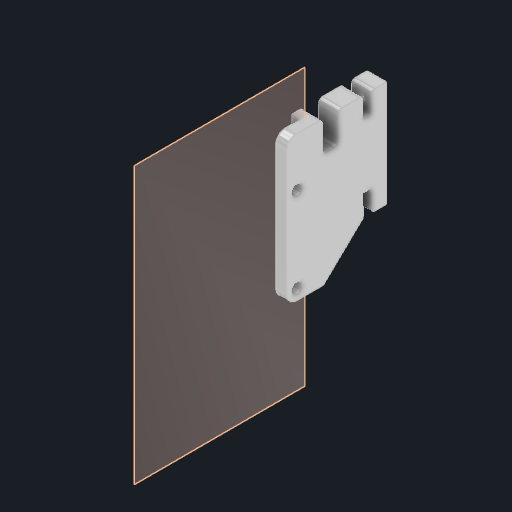
# Autodesk Inventor part: Dynamixel Vertical fixation
Saved by Autodesk Inventor 2024.3 (Build 283343000, 343)
## iProperties
Created: 2022-06-18
Part Number: Dynamixel Vertical fixation
Material: 알루미늄 6061
Document SubType Name: Sheet Metal
Designer: 박지훈
Density: 2.7 g/cm^3
Sheet Metal Rule: 기본값_mm
Appearance: 알루미늄 - 연마
Flat Pattern Width: 0.5 cm
Flat Pattern Length: 3.74 cm
Flat Pattern Area: 1.87 cm^2
Sheet Metal Width: 5.000 mm
Sheet Metal Length: 37.400 mm
Sheet Metal Area: 187.000 mm^2
Author: 박지훈
Autodesk Inventor part; units mm, degrees
ref_plane "YZ Plane" through (0, 0, 0) normal (1, 0, 0) x (0, 1, 0)
ref_plane "XZ Plane" through (0, 0, 0) normal (0, 1, 0) x (-1, 0, 0)
ref_plane "XY Plane" through (0, 0, 0) normal (0, 0, 1) x (1, 0, 0)
ref_plane "작업 평면1" through (19.4452, -233.7171, 54.1562) normal (1, 0, 0) x (0, 0, 1)
sketch "스케치1" plane through (19.4452, -233.7171, 54.1562) normal (1, 0, 0) x (0, 0, 1)
  line L0 (-15, 14.5) -> (-11.5, 14.5) projected
  line L1 (-15, 14.5) -> (-20.1, 8.5) projected
  line L2 (-20.1, 8.5) -> (-20.1, -44.6) projected
  line L3 (-20.1, -44.6) -> (-15, -50.6) projected
  line L4 (-15, -50.6) -> (15, -50.6) projected
  line L5 (15, -50.6) -> (20.1, -44.6) projected
  line L6 (20.1, -44.6) -> (20.1, 8.5) projected
  line L7 (20.1, 8.5) -> (15, 14.5) projected
  line L8 (11.5, 14.5) -> (15, 14.5) projected
  arc A0 (14.5, 11.5) -> (11.5, 14.5) centre (11.5, 11.5) ccw projected
  line L9 (14.5, -42) -> (14.5, 11.5) projected
  arc A1 (11.5, -45) -> (14.5, -42) centre (11.5, -42) ccw projected
  line L10 (-11.5, -45) -> (11.5, -45) projected
  arc A2 (-14.5, -42) -> (-11.5, -45) centre (-11.5, -42) ccw projected
  line L11 (-14.5, 11.5) -> (-14.5, -42) projected
  arc A3 (-11.5, 14.5) -> (-14.5, 11.5) centre (-11.5, 11.5) ccw projected
  circle A4 centre (-17.3, 4) radius 1.35 projected
  circle A5 centre (-17.3, -18) radius 1.35 projected
  circle A6 centre (-11, -47.8) radius 1.35 projected
  circle A7 centre (17.3, 4) radius 1.35 projected
  circle A8 centre (17.3, -18) radius 1.35 projected
  circle A9 centre (11, -47.8) radius 1.35 projected
  circle A10 centre (-17.3, -40) radius 1.35 projected
  circle A11 centre (17.3, -40) radius 1.35 projected
  line L12 (-14.9538, -50.5) -> (-20, -44.5632)
  line L13 (-20, 8.4632) -> (-14.9538, 14.4)
  line L14 (-14.9538, 14.4) -> (-12.5954, 14.4)
  arc A12 (-12.5954, 14.4) -> (-14.6, 11.5) centre (-11.5, 11.5) ccw
  line L15 (-14.6, 11.5) -> (-14.6, -42)
  arc A13 (-14.6, -42) -> (-11.5, -45.1) centre (-11.5, -42) ccw
  line L16 (-11.5, -45.1) -> (11.5, -45.1)
  arc A14 (11.5, -45.1) -> (14.6, -42) centre (11.5, -42) ccw
  line L17 (14.6, -42) -> (14.6, 11.5)
  arc A15 (14.6, 11.5) -> (12.5954, 14.4) centre (11.5, 11.5) ccw
  line L18 (12.5954, 14.4) -> (14.9538, 14.4)
  line L19 (14.9538, 14.4) -> (20, 8.4632)
  line L20 (20, 8.4632) -> (20, -44.5632)
  line L21 (20, -44.5632) -> (14.9538, -50.5)
  line L22 (14.9538, -50.5) -> (-14.9538, -50.5)
  arc A16 (-17.3, -42.7) -> (-14.6, -40) centre (-17.3, -40) ccw
  arc A17 (-14.6, -18) -> (-17.3, -15.3) centre (-17.3, -18) ccw
  line L23 (-17.3, -42.7) -> (-36.1, -42.7)
  line L24 (-36.1, -15.3) -> (-17.3, -15.3)
  line L25 (-36.1, -40) -> (-36.1, -37.3)
  line L26 (-36.1, -37.3) -> (-20.2, -37.3)
  line L27 (-36.1, -18) -> (-36.1, -20.7)
  line L28 (-20, -44.5632) -> (-20, -42.7)
  line L29 (-20, -15.3) -> (-20, 8.4632)
  line L30 (-36.1, -42.7) -> (-36.1, -37.3)
  line L31 (-36.1, -20.7) -> (-36.1, -15.3)
  line L32 (-20.2, -37.3) -> (-20.2, -20.7)
  line L33 (-36.1, -20.7) -> (-20.2, -20.7)
  point P0 (-36.1, -40)
  point P1 (-36.1, -18)
  dimension "d0" = 0.1
  dimension "d1" = 18.8
  dimension "d2" = 2.7
  dimension "d3" = 2.7
  constraints: 44 end point, 12 point on circle, 6 centre point, 4 point on line, 2 coincident, 2 perpendicular, 2 tangent, 1 horizontal, 1 parallel, 13 other
  measures "d0" distance between parallel lines of L3 L12
  measures "d1" distance of L24.end L24.start
  measures "d2" distance of L25.start L25.end
  measures "d3" distance of L27.end L27.start
extrude "돌출1" add sketch "스케치1" along normal blind 2.75 contours L24 A17 L15 A16 L23 L2 | L2 L23 L30 L25 L26 L32 L33 L27 L31 L24
sketch "스케치2" plane through (19.4452, -233.7171, 54.1562) normal (-1, 0, 0) x (0, 0, 1)
  line L0 (-36.1, 37.3) -> (-36.1, 42.7) projected
  line L1 (-20.2, 37.3) -> (-36.1, 37.3) projected
  line L2 (-20.2, 20.7) -> (-20.2, 37.3) projected
  line L3 (-36.1, 20.7) -> (-20.2, 20.7) projected
  line L4 (-36.1, 15.3) -> (-36.1, 20.7) projected
  line L5 (-17.3, 15.3) -> (-36.1, 15.3) projected
  arc A0 (-17.3, 15.3) -> (-14.6, 18) centre (-17.3, 18) ccw projected
  line L6 (-14.6, 40) -> (-14.6, 18) projected
  arc A1 (-14.6, 40) -> (-17.3, 42.7) centre (-17.3, 40) ccw projected
  line L7 (-36.1, 42.7) -> (-17.3, 42.7) projected
  circle A2 centre (-17.3, 40) radius 1.35 projected
  circle A3 centre (-17.3, 18) radius 1.35 projected
  line L8 (-36.1, 37.3) -> (-36.1, 42.7) projected
  line L9 (-36.1, 42.7) -> (-17.3, 42.7) projected
  line L10 (-36.1, 37.3) -> (-20.2, 37.3)
  line L11 (-20.2, 37.3) -> (-20.2, 42.7)
  line L12 (-20.2, 42.7) -> (-36.1, 42.7)
  line L13 (-36.1, 42.7) -> (-36.1, 37.3)
  line L14 (-36.1, 20.7) -> (-20.2, 20.7) projected
  line L15 (-17.3, 15.3) -> (-36.1, 15.3) projected
  line L16 (-20.2, 20.7) -> (-36.1, 20.7)
  line L17 (-36.1, 20.7) -> (-36.1, 15.3)
  line L18 (-36.1, 15.3) -> (-20.2, 15.3)
  line L19 (-20.2, 15.3) -> (-20.2, 20.7)
  point P0 (-20.2, 15.3)
  point P1 (-20.2, 37.3)
  point P2 (-20.2, 42.7)
  constraints: 16 end point, 4 parallel, 2 horizontal, 2 perpendicular, 1 point on line
extrude "돌출2" add sketch "스케치2" along normal blind 2.25 contours L0 L7 L11 L1 | L19 L5 L4 L3
sketch "스케치3" plane through (22.1952, -196.4171, 18.0562) normal (0, 0, -1) x (-1, 0, 0)
  line L0 (5, 5.4) -> (0, 5.4) projected
  line L1 (0, 0) -> (0, 5.4) projected
  line L2 (0, 0) -> (5, 0) projected
  line L3 (5, 5.4) -> (5, 0) projected
  line L4 (5, -16.6) -> (0, -16.6) projected
  line L5 (0, -22) -> (0, -16.6) projected
  line L6 (5, -22) -> (0, -22) projected
  line L7 (5, -16.6) -> (5, -22) projected
  line L8 (0, 0) -> (5, 0) projected
  line L9 (2.75, 2.7) -> (0, 2.7) projected
  line L10 (5, 0) -> (2.5, 0)
  line L11 (2.5, 0) -> (2.5, 2.7)
  line L12 (2.5, 2.7) -> (5, 2.7)
  line L13 (5, 2.7) -> (5, 0)
  circle A0 centre (2.5, 2.7) radius 1
  line L14 (2.75, -19.3) -> (0, -19.3) projected
  circle A1 centre (2.5, -19.3) radius 1
  dimension "d9" = 2
  dimension "d10" = 2
  constraints: 8 end point, 2 centre point, 2 parallel, 2 point on line, 1 coincident, 1 horizontal, 1 perpendicular
  measures "d9" diameter of A0
  measures "d10" diameter of A1
extrude "돌출3" cut sketch "스케치3" against normal blind 10 contours A0 L11 L9 L12 | L12 L9 A0 | L9 L11 A0 | A1
sketch "스케치4" plane through (22.1952, -196.4171, 18.0562) normal (0, 0, -1) x (-1, 0, 0)
  circle A0 centre (2.5, 2.7) radius 1 projected
  line L0 (5, 5.4) -> (0, 5.4) projected
  line L1 (0, 0) -> (0, 5.4) projected
  line L2 (0, 0) -> (5, 0) projected
  line L3 (5, 5.4) -> (5, 0) projected
  circle A1 centre (2.5, -19.3) radius 1 projected
  line L4 (5, -16.6) -> (0, -16.6) projected
  line L5 (0, -22) -> (0, -16.6) projected
  line L6 (5, -22) -> (0, -22) projected
  line L7 (5, -16.6) -> (5, -22) projected
extrude "돌출4" cut sketch "스케치4" against normal blind 1.7
sketch "스케치5" plane through (22.1952, -196.4171, 19.7562) normal (0, 0, -1) x (-1, 0, 0)
  line L0 (5, 5.4) -> (5, 0) projected
  line L1 (0, 5.4) -> (5, 5.4) projected
  line L2 (0, 0) -> (0, 5.4) projected
  line L3 (5, 0) -> (0, 0) projected
  circle A0 centre (2.5, 2.7) radius 1 projected
  line L4 (0, -16.6) -> (5, -16.6) projected
  line L5 (0, -22) -> (0, -16.6) projected
  line L6 (5, -22) -> (0, -22) projected
  line L7 (5, -16.6) -> (5, -22) projected
  circle A1 centre (2.5, -19.3) radius 1 projected
extrude "돌출5" add sketch "스케치5" along normal blind 0.6
sketch "스케치6" plane through (22.1952, -196.4171, 19.1562) normal (0, 0, -1) x (-1, 0, 0)
  line L0 (0, 5.4) -> (0, 0) projected
  line L1 (0, 0) -> (5, 0) projected
  line L2 (5, 0) -> (5, 5.4) projected
  line L3 (5, 5.4) -> (0, 5.4) projected
  circle A0 centre (2.5, 2.7) radius 1 projected
  line L4 (0, -22) -> (5, -22) projected
  line L5 (5, -22) -> (5, -16.6) projected
  line L6 (5, -16.6) -> (0, -16.6) projected
  line L7 (0, -16.6) -> (0, -22) projected
  circle A1 centre (2.5, -19.3) radius 1 projected
extrude "돌출6" cut sketch "스케치6" against normal blind 2.5 contours L3 L2 L1 L0 | A0 | L7 L6 L5 L4
sketch "스케치7" plane through (22.1952, -196.4171, 21.6562) normal (0, 0, -1) x (-1, 0, 0)
  line L0 (5, -16.6) -> (5, -22) projected
  line L1 (0, -16.6) -> (5, -16.6) projected
  line L2 (0, -22) -> (0, -16.6) projected
  line L3 (5, -22) -> (0, -22) projected
  circle A0 centre (2.5, -19.3) radius 1 projected
  circle A1 centre (2.5, 2.7) radius 1 projected
  line L4 (5, 0) -> (0, 0) projected
  line L5 (5, 5.4) -> (5, 0) projected
  line L6 (0, 5.4) -> (5, 5.4) projected
  line L7 (0, 0) -> (0, 5.4) projected
extrude "돌출7" add sketch "스케치7" along normal blind 0.2
sketch "스케치8" plane through (22.1952, -196.4171, 21.4562) normal (0, 0, -1) x (-1, 0, 0)
  line L0 (5, 5.4) -> (0, 5.4) projected
  line L1 (0, 5.4) -> (0, 0) projected
  line L2 (0, 0) -> (5, 0) projected
  line L3 (5, 0) -> (5, 5.4) projected
  circle A0 centre (2.5, 2.7) radius 1 projected
  line L4 (0, -16.6) -> (0, -22) projected
  line L5 (0, -22) -> (5, -22) projected
  line L6 (5, -22) -> (5, -16.6) projected
  line L7 (5, -16.6) -> (0, -16.6) projected
  circle A1 centre (2.5, -19.3) radius 1 projected
  point P0 (22.1952, 196.4171)
extrude "돌출8" add sketch "스케치8" along normal blind 1.3
move faces "이동1" translate (0, 0, -6.5) faces at (19.7354, -217.848, 20.1562) (19.7354, -191.5861, 20.1562)
sketch "스케치9" plane through (22.1952, -233.7171, 54.1562) normal (1, 0, 0) x (0, 0, -1)
  line L0 (40.5, 20.7) -> (20.2, 20.7) projected
  line L1 (20.2, 20.7) -> (20.2, 37.3) projected
  line L2 (20.2, 37.3) -> (40.5, 37.3) projected
  line L3 (40.5, 42.7) -> (40.5, 37.3) projected
  line L4 (40.5, 42.7) -> (17.3, 42.7) projected
  arc A0 (17.3, 42.7) -> (14.6, 40) centre (17.3, 40) ccw projected
  line L5 (14.6, 40) -> (14.6, 18) projected
  arc A1 (14.6, 18) -> (17.3, 15.3) centre (17.3, 18) ccw projected
  line L6 (17.3, 15.3) -> (40.5, 15.3) projected
  line L7 (40.5, 20.7) -> (40.5, 15.3) projected
  circle A2 centre (17.3, 40) radius 1.35 projected
  circle A3 centre (17.3, 18) radius 1.35 projected
  line L8 (40.5, 42.7) -> (40.5, 15.3)
  line L9 (30.5, 42.7) -> (30.5, 15.3)
  point P0 (54.1562, 233.7171)
  point P1 (30.5, 37.3)
  point P2 (30.5, 20.7)
  point P3 (40.5, 20.7)
  dimension "d26" = 10
  constraints: 4 end point, 1 collinear, 1 parallel
  measures "d26" distance between parallel lines of L8 L9
extrude "돌출9" add sketch "스케치9" against normal up to surface (5 mm away) contours L0 L9 L2 L8
sketch "스케치10" plane through (22.1952, -233.7171, 54.1562) normal (1, 0, 0) x (0, 0, -1)
  line L0 (30.5, 20.7) -> (20.2, 20.7) projected
  line L1 (20.2, 20.7) -> (20.2, 37.3) projected
  line L2 (20.2, 37.3) -> (30.5, 37.3) projected
  line L3 (30.5, 37.3) -> (30.5, 20.7) projected
  line L4 (40.5, 42.7) -> (40.5, 15.3) projected
  line L5 (40.5, 42.7) -> (17.3, 42.7) projected
  arc A0 (17.3, 42.7) -> (14.6, 40) centre (17.3, 40) ccw projected
  line L6 (14.6, 40) -> (14.6, 18) projected
  arc A1 (14.6, 18) -> (17.3, 15.3) centre (17.3, 18) ccw projected
  line L7 (17.3, 15.3) -> (40.5, 15.3) projected
  circle A2 centre (17.3, 40) radius 1.35 projected
  circle A3 centre (17.3, 18) radius 1.35 projected
  line L8 (40.5, 42.7) -> (40.5, 15.3)
  line L9 (40.5, 15.3) -> (30.5, 15.3)
  line L10 (30.5, 15.3) -> (30.5, 42.7)
  line L11 (30.5, 42.7) -> (40.5, 42.7)
  point P0 (54.1562, 233.7171)
  point P1 (30.5, 42.7)
  point P2 (30.5, 15.3)
  constraints: 8 end point, 3 equal length, 1 perpendicular
extrude "돌출10" cut sketch "스케치10" against normal through all contours L10 L7 A1 L6 A0 L5 L2 L1 L0
sketch "스케치11" plane through (22.1952, -233.7171, 54.1562) normal (1, 0, 0) x (0, 0, -1)
  line L0 (-15, 62.5) -> (-11.5, 62.5) projected
  line L1 (-15, 62.5) -> (-20.1, 56.5) projected
  line L2 (-20.1, 56.5) -> (-20.1, 3.4) projected
  line L3 (-20.1, 3.4) -> (-15, -2.6) projected
  line L4 (-15, -2.6) -> (15, -2.6) projected
  line L5 (15, -2.6) -> (20.1, 3.4) projected
  line L6 (20.1, 3.4) -> (20.1, 56.5) projected
  line L7 (20.1, 56.5) -> (15, 62.5) projected
  line L8 (11.5, 62.5) -> (15, 62.5) projected
  arc A0 (14.5, 59.5) -> (11.5, 62.5) centre (11.5, 59.5) ccw projected
  line L9 (14.5, 6) -> (14.5, 59.5) projected
  arc A1 (11.5, 3) -> (14.5, 6) centre (11.5, 6) ccw projected
  line L10 (-11.5, 3) -> (11.5, 3) projected
  arc A2 (-14.5, 6) -> (-11.5, 3) centre (-11.5, 6) ccw projected
  line L11 (-14.5, 59.5) -> (-14.5, 6) projected
  arc A3 (-11.5, 62.5) -> (-14.5, 59.5) centre (-11.5, 59.5) ccw projected
  circle A4 centre (17.3, 52) radius 1.35 projected
  circle A5 centre (17.3, 30) radius 1.35 projected
  circle A6 centre (17.3, 8) radius 1.35 projected
  circle A7 centre (11, 0.2) radius 1.35 projected
  circle A8 centre (-17.3, 52) radius 1.35 projected
  circle A9 centre (-17.3, 30) radius 1.35 projected
  circle A10 centre (-17.3, 8) radius 1.35 projected
  circle A11 centre (-11, 0.2) radius 1.35 projected
  line L12 (17.3, 30) -> (17.3, 8) construction
  line L13 (14.6, 30) -> (14.6, 8)
  line L14 (20, 8) -> (20, 30)
  arc A12 (20, 30) -> (14.6, 30) centre (17.3, 30) ccw
  arc A13 (14.6, 8) -> (20, 8) centre (17.3, 8) ccw
  line L15 (17.3, 32.7) -> (17.3, 5.3)
  line L16 (17.3, 5.3) -> (24.3, 5.3)
  line L17 (24.3, 5.3) -> (24.3, 32.7)
  line L18 (24.3, 32.7) -> (17.3, 32.7)
  line L19 (24.3, 32.7) -> (30.5, 42.7)
  line L20 (40.5, 15.3) -> (30.5, 15.3) projected
  line L21 (24.3, 5.3) -> (30.5, 15.3)
  line L22 (30.5, 42.7) -> (30.5, 15.3) projected
  line L23 (30.5, 15.3) -> (40.5, 15.3) projected
  line L24 (40.5, 42.7) -> (40.5, 15.3) projected
  line L25 (40.5, 42.7) -> (30.5, 42.7) projected
  point P0 (54.1562, 233.7171)
  point P1 (17.3, 19)
  point P2 (30.5, 42.7)
  dimension "d31" = 5.4
  dimension "d32" = 7
  constraints: 20 end point, 6 point on circle, 4 tangent, 3 parallel, 2 centre point, 1 midpoint, 1 perpendicular, 1 vertical
  measures "d31" diameter of A13
  measures "d32" distance of L16.end L15.end
extrude "돌출11" add sketch "스케치11" against normal blind 2.75 contours L16 A13 L14 A12 L18 L6 | L6 L18 L17 L16 | L15 A6 A5 A12 L14 A13 | A13 L13 A12 L15 A5 A6 | L17 L19 L22 L21
sketch "스케치12" plane through (19.4452, -233.7171, 54.1562) normal (-1, 0, 0) x (0, 0, 1)
  line L0 (-14.6, 8) -> (-14.6, 30) projected
  arc A0 (-14.6, 30) -> (-17.3, 32.7) centre (-17.3, 30) ccw projected
  line L1 (-17.3, 32.7) -> (-24.3, 32.7) projected
  line L2 (-24.3, 32.7) -> (-30.5, 42.7) projected
  line L3 (-30.5, 40.9682) -> (-30.5, 42.7) projected
  line L4 (-30.5, 40.9682) -> (-30.5, 39.0318) projected
  line L5 (-30.5, 18.9682) -> (-30.5, 39.0318) projected
  line L6 (-30.5, 18.9682) -> (-30.5, 17.0318) projected
  line L7 (-30.5, 15.3) -> (-30.5, 17.0318) projected
  line L8 (-30.5, 15.3) -> (-24.3, 5.3) projected
  line L9 (-24.3, 5.3) -> (-17.3, 5.3) projected
  arc A1 (-17.3, 5.3) -> (-14.6, 8) centre (-17.3, 8) ccw projected
  circle A2 centre (-17.3, 30) radius 1.35 projected
  circle A3 centre (-17.3, 8) radius 1.35 projected
  line L10 (13.5, 8.25) -> (11.5, 8.25) projected
  arc A4 (11.5, 8.25) -> (9.25, 6) centre (11.5, 6) ccw projected
  line L11 (9.25, 6) -> (9.25, 4) projected
  arc A5 (8.25, 3) -> (9.25, 4) centre (8.25, 4) ccw projected
  line L12 (8.25, 3) -> (-8.25, 3) projected
  arc A6 (-9.25, 4) -> (-8.25, 3) centre (-8.25, 4) ccw projected
  line L13 (-9.25, 4) -> (-9.25, 6) projected
  arc A7 (-9.25, 6) -> (-11.5, 8.25) centre (-11.5, 6) ccw projected
  line L14 (-11.5, 8.25) -> (-13.5, 8.25) projected
  arc A8 (-14.5, 9.25) -> (-13.5, 8.25) centre (-13.5, 9.25) ccw projected
  line L15 (-14.5, 9.25) -> (-14.5, 56.25) projected
  arc A9 (-13.5, 57.25) -> (-14.5, 56.25) centre (-13.5, 56.25) ccw projected
  line L16 (-13.5, 57.25) -> (-11.5, 57.25) projected
  arc A10 (-11.5, 57.25) -> (-9.25, 59.5) centre (-11.5, 59.5) ccw projected
  line L17 (-9.25, 59.5) -> (-9.25, 62.5) projected
  line L18 (-15, 62.5) -> (-9.25, 62.5) projected
  line L19 (-20.1, 56.5) -> (-15, 62.5) projected
  line L20 (-20.1, 3.4) -> (-20.1, 56.5) projected
  line L21 (-15, -2.6) -> (-20.1, 3.4) projected
  line L22 (15, -2.6) -> (-15, -2.6) projected
  line L23 (20.1, 3.4) -> (15, -2.6) projected
  line L24 (20.1, 56.5) -> (20.1, 3.4) projected
  line L25 (15, 62.5) -> (20.1, 56.5) projected
  line L26 (9.25, 62.5) -> (15, 62.5) projected
  line L27 (9.25, 62.5) -> (9.25, 59.5) projected
  arc A11 (9.25, 59.5) -> (11.5, 57.25) centre (11.5, 59.5) ccw projected
  line L28 (11.5, 57.25) -> (13.5, 57.25) projected
  arc A12 (14.5, 56.25) -> (13.5, 57.25) centre (13.5, 56.25) ccw projected
  line L29 (14.5, 56.25) -> (14.5, 9.25) projected
  arc A13 (13.5, 8.25) -> (14.5, 9.25) centre (13.5, 9.25) ccw projected
  circle A14 centre (17.3, 52) radius 1.35 projected
  circle A15 centre (17.3, 30) radius 1.35 projected
  circle A16 centre (11, 0.2) radius 1.35 projected
  circle A17 centre (-17.3, 52) radius 1.35 projected
  circle A18 centre (-17.3, 30) radius 1.35 projected
  circle A19 centre (-11, 0.2) radius 1.35 projected
  circle A20 centre (17.3, 8) radius 1.35 projected
  circle A21 centre (-17.3, 8) radius 1.35 projected
  line L30 (-21.1, 56.8676) -> (-15.4624, 63.5)
  line L31 (-15.4624, 63.5) -> (-8.25, 63.5)
  line L32 (-8.25, 63.5) -> (-8.25, 59.5)
  arc A22 (-11.5, 56.25) -> (-8.25, 59.5) centre (-11.5, 59.5) ccw
  line L33 (-11.5, 56.25) -> (-13.5, 56.25)
  line L34 (-13.5, 56.25) -> (-13.5, 9.25)
  line L35 (-13.5, 9.25) -> (-11.5, 9.25)
  arc A23 (-8.25, 6) -> (-11.5, 9.25) centre (-11.5, 6) ccw
  line L36 (-8.25, 6) -> (-8.25, 4)
  line L37 (-8.25, 4) -> (8.25, 4)
  line L38 (8.25, 4) -> (8.25, 6)
  arc A24 (11.5, 9.25) -> (8.25, 6) centre (11.5, 6) ccw
  line L39 (11.5, 9.25) -> (13.5, 9.25)
  line L40 (13.5, 9.25) -> (13.5, 56.25)
  line L41 (13.5, 56.25) -> (11.5, 56.25)
  arc A25 (8.25, 59.5) -> (11.5, 56.25) centre (11.5, 59.5) ccw
  line L42 (8.25, 59.5) -> (8.25, 63.5)
  line L43 (8.25, 63.5) -> (15.4624, 63.5)
  line L44 (15.4624, 63.5) -> (21.1, 56.8676)
  line L45 (21.1, 56.8676) -> (21.1, 3.0324)
  line L46 (21.1, 3.0324) -> (15.4624, -3.6)
  line L47 (15.4624, -3.6) -> (-15.4624, -3.6)
  line L48 (-15.4624, -3.6) -> (-21.1, 3.0324)
  line L49 (-21.1, 3.0324) -> (-21.1, 56.8676)
  point P0 (-54.1562, 233.7171)
  point P1 (-21.1, 5.3)
  point P2 (-21.1, 32.7)
  dimension "d35" = 1
  constraints: 40 end point, 8 point on circle, 4 centre point, 23 other
  measures "d35" distance between parallel lines of L20 L49
extrude "돌출12" add sketch "스케치12" along normal up to surface (2.25 mm away) contours L9 L8 L7 L6 L5 L4 L3 L2 L1 L49
fillet "모깎기1" radius 5 3 edges at (19.6952, -218.4171, 23.6562) (19.6952, -191.0171, 23.6562) (19.6952, -201.0171, 29.8562)
sketch "스케치13" plane through (22.1952, -233.7171, 54.1562) normal (1, 0, 0) x (0, 0, -1)
  arc A0 (33.283, 42.7) -> (29.0335, 40.3347) centre (33.283, 37.7) ccw projected
  line L0 (29.0335, 40.3347) -> (25.7665, 35.0653) projected
  arc A1 (21.517, 32.7) -> (25.7665, 35.0653) centre (21.517, 37.7) ccw projected
  line L1 (21.517, 32.7) -> (17.3, 32.7) projected
  arc A2 (17.3, 32.7) -> (14.6, 30) centre (17.3, 30) ccw projected
  line L2 (14.6, 30) -> (14.6, 8) projected
  arc A3 (14.6, 8) -> (17.3, 5.3) centre (17.3, 8) ccw projected
  line L3 (17.3, 5.3) -> (24.3, 5.3) projected
  line L4 (24.3, 5.3) -> (29.0335, 12.9347) projected
  arc A4 (33.283, 15.3) -> (29.0335, 12.9347) centre (33.283, 10.3) ccw projected
  line L5 (33.283, 15.3) -> (40.5, 15.3) projected
  line L6 (40.5, 42.7) -> (40.5, 15.3) projected
  line L7 (40.5, 42.7) -> (33.283, 42.7) projected
  circle A5 centre (17.3, 30) radius 1.35 projected
  circle A6 centre (17.3, 8) radius 1.35 projected
  line L8 (30.8659, 31.9037) -> (33.8396, 36.7)
  line L9 (33.8396, 36.7) -> (34.5, 36.7)
  line L10 (34.5, 36.7) -> (34.5, 21.3)
  line L11 (34.5, 21.3) -> (33.283, 21.3)
  arc A7 (33.283, 21.3) -> (23.9341, 16.0963) centre (33.283, 10.3) ccw
  line L12 (23.9341, 16.0963) -> (20.9604, 11.3)
  line L13 (20.9604, 11.3) -> (20.6, 11.3)
  line L14 (20.6, 11.3) -> (20.6, 26.7)
  line L15 (20.6, 26.7) -> (21.517, 26.7)
  arc A8 (21.517, 26.7) -> (30.8659, 31.9037) centre (21.517, 37.7) ccw
  point P0 (54.1562, 233.7171)
  dimension "d39" = 6
  constraints: 16 end point, 4 point on circle, 2 centre point, 9 other
  measures "d39" radial gap between concentric circles of A1 A8
extrude "돌출13" cut sketch "스케치13" against normal through all contours L8 L9 L10 L11 A7 L12 L13 L14 L15 A8
fillet "모깎기2" radius 1 6 edges at (19.6952, -197.0171, 19.6562) (19.6952, -197.0171, 20.3166) (19.6952, -212.4171, 19.6562) (20.8202, -222.4171, 33.1958) (20.8202, -222.4171, 33.5562) (20.8202, -207.0171, 33.5562)
sketch "스케치14" plane through (22.1952, -233.7171, 54.1562) normal (1, 0, 0) x (0, 0, -1)
  line L0 (34.5, 34.2545) -> (34.5, 22.3) projected
  arc A0 (33.5, 21.3) -> (34.5, 22.3) centre (33.5, 22.3) ccw projected
  line L1 (33.5, 21.3) -> (33.283, 21.3) projected
  arc A1 (33.283, 21.3) -> (23.9341, 16.0963) centre (33.283, 10.3) ccw projected
  line L2 (23.9341, 16.0963) -> (22.4499, 13.7025) projected
  arc A2 (20.6, 14.2294) -> (22.4499, 13.7025) centre (21.6, 14.2294) ccw projected
  line L3 (20.6, 14.2294) -> (20.6, 25.7003) projected
  arc A3 (21.5931, 26.7003) -> (20.6, 25.7003) centre (21.6, 25.7003) ccw projected
  arc A4 (21.5931, 26.7003) -> (30.8659, 31.9037) centre (21.517, 37.7) ccw projected
  line L4 (30.8659, 31.9037) -> (32.6501, 34.7814) projected
  arc A5 (34.5, 34.2545) -> (32.6501, 34.7814) centre (33.5, 34.2545) ccw projected
  arc A6 (33.283, 42.7) -> (29.0335, 40.3347) centre (33.283, 37.7) ccw projected
  line L5 (29.0335, 40.3347) -> (25.7665, 35.0653) projected
  arc A7 (21.517, 32.7) -> (25.7665, 35.0653) centre (21.517, 37.7) ccw projected
  line L6 (21.517, 32.7) -> (17.3, 32.7) projected
  arc A8 (17.3, 32.7) -> (14.6, 30) centre (17.3, 30) ccw projected
  line L7 (14.6, 30) -> (14.6, 8) projected
  arc A9 (14.6, 8) -> (17.3, 5.3) centre (17.3, 8) ccw projected
  line L8 (17.3, 5.3) -> (24.3, 5.3) projected
  line L9 (24.3, 5.3) -> (29.0335, 12.9347) projected
  arc A10 (33.283, 15.3) -> (29.0335, 12.9347) centre (33.283, 10.3) ccw projected
  line L10 (33.283, 15.3) -> (40.5, 15.3) projected
  line L11 (40.5, 42.7) -> (40.5, 15.3) projected
  line L12 (40.5, 42.7) -> (33.283, 42.7) projected
  circle A11 centre (17.3, 30) radius 1.35 projected
  circle A12 centre (17.3, 8) radius 1.35 projected
  line L13 (14.6, 30) -> (14.6, 8) projected
  line L14 (14.6, 30) -> (40.5, 30)
  line L15 (40.5, 30) -> (40.5, 42.7)
  line L16 (40.5, 42.7) -> (14.6, 42.7)
  line L17 (14.6, 42.7) -> (14.6, 30)
  line L18 (24.3, 5.3) -> (40.5, 5.3)
  line L19 (40.5, 5.3) -> (40.5, 15.3)
  line L20 (40.5, 15.3) -> (24.3, 15.3)
  line L21 (24.3, 15.3) -> (24.3, 5.3)
  point P0 (54.1562, 233.7171)
  constraints: 16 end point, 4 parallel, 2 horizontal, 2 perpendicular
extrude "돌출14" add sketch "스케치14" against normal up to surface (2.75 mm away) contours L0 L14 A4 L4 A5 | L0 A0 L1 A1 L2 A2 L3 A3 A4 L14 | L19 L18 L9 A10 L10 | A6 L5 A7 L6 A8 L17 L16
sketch "스케치15" plane through (19.4452, -228.4171, 13.6562) normal (-1, 0, 0) x (0, 0, 1)
  arc A0 (11.4665, 7.6347) -> (7.217, 10) centre (7.217, 5) ccw projected
  line L0 (0, 10) -> (7.217, 10) projected
  line L1 (0, 10) -> (0, 0) projected
  line L2 (0, 0) -> (16.2, 0) projected
  line L3 (11.4665, 7.6347) -> (16.2, 0) projected
  line L4 (0, 37.4) -> (25.9, 37.4) projected
  line L5 (25.9, 37.4) -> (25.9, 2.7) projected
  arc A1 (23.2, 0) -> (25.9, 2.7) centre (23.2, 2.7) ccw projected
  line L6 (23.2, 0) -> (0, 0) projected
  line L7 (0, 37.4) -> (0, 0) projected
  circle A2 centre (23.2, 24.7) radius 1.35 projected
  circle A3 centre (23.2, 2.7) radius 1.35 projected
  line L8 (19.4, 8.0634) -> (19.4, 0) projected
  line L9 (19.4, 0) -> (23.2, 0) projected
  arc A4 (23.2, 0) -> (25.9, 2.7) centre (23.2, 2.7) ccw projected
  line L10 (25.9, 2.7) -> (25.9, 37.4) projected
  line L11 (25.9, 37.4) -> (7.217, 37.4) projected
  arc A5 (11.4665, 35.0347) -> (7.217, 37.4) centre (7.217, 32.4) ccw projected
  line L12 (14.7335, 29.7653) -> (11.4665, 35.0347) projected
  arc A6 (14.7335, 29.7653) -> (18.983, 27.4) centre (18.983, 32.4) ccw projected
  line L13 (19.4, 27.4) -> (18.983, 27.4) projected
  line L14 (19.4, 27.4) -> (19.4, 21.2663) projected
  arc A7 (19.4, 21.2663) -> (18.9069, 21.4003) centre (18.9, 20.4003) ccw projected
  arc A8 (18.0501, 8.4025) -> (19.4, 8.0634) centre (18.9, 8.9294) ccw projected
  circle A9 centre (23.2, 2.7) radius 1.35 projected
  circle A10 centre (23.2, 24.7) radius 1.35 projected
  line L15 (19.4, 8.0634) -> (19.4, 0) projected
  line L16 (0, 37.4) -> (25.9, 37.4) projected
  line L17 (19.4, 0) -> (25.9, 0)
  line L18 (25.9, 0) -> (25.9, 37.4)
  line L19 (25.9, 37.4) -> (19.4, 37.4)
  line L20 (19.4, 37.4) -> (19.4, 0)
  arc A11 (9.6341, 26.6037) -> (18.9069, 21.4003) centre (18.983, 32.4) ccw projected
  line L21 (7.8499, 29.4814) -> (9.6341, 26.6037) projected
  arc A12 (7.8499, 29.4814) -> (6, 28.9545) centre (7, 28.9545) ccw projected
  line L22 (6, 17) -> (6, 28.9545) projected
  arc A13 (6, 17) -> (7, 16) centre (7, 17) ccw projected
  line L23 (7.217, 16) -> (7, 16) projected
  arc A14 (16.5659, 10.7963) -> (7.217, 16) centre (7.217, 5) ccw projected
  line L24 (18.0501, 8.4025) -> (16.5659, 10.7963) projected
  point P0 (-13.6562, 228.4171)
  point P1 (19.4, 37.4)
  point P2 (7.217, 37.4)
  constraints: 8 end point, 2 parallel, 1 horizontal, 1 perpendicular
extrude "돌출15" add sketch "스케치15" along normal up to surface (2.25 mm away) contours L3 L2 L1 L0 A0 | A8 L24 A14 L23 A13 L22 A12 L21 A11 A7 L20 | L4 L20 L13 A6 L12 A5
fillet "모깎기3" radius 2.5 1 edges at (20.8202, -191.0171, 39.5562)
sketch "스케치16" plane through (22.1952, -233.7171, 54.1562) normal (1, 0, 0) x (0, 0, -1)
  circle A0 centre (17.3, 8) radius 1.35 projected
  circle A1 centre (17.3, 30) radius 1.35 projected
  arc A2 (17.1, 42.7) -> (14.6, 40.2) centre (17.1, 40.2) ccw projected
  line L0 (14.6, 40.2) -> (14.6, 8) projected
  arc A3 (14.6, 8) -> (17.3, 5.3) centre (17.3, 8) ccw projected
  line L1 (17.3, 5.3) -> (40.5, 5.3) projected
  line L2 (40.5, 42.7) -> (40.5, 5.3) projected
  line L3 (40.5, 42.7) -> (17.1, 42.7) projected
  line L4 (24.5, 46.4593) -> (24.5, 81.4701) projected
  line L5 (27.5, 81.4701) -> (27.5, 46.4593) projected
  line L6 (24.5, 81.4701) -> (27.5, 81.4701)
  line L7 (27.5, 81.4701) -> (27.5, 42.7)
  line L8 (27.5, 42.7) -> (24.5, 42.7)
  line L9 (24.5, 42.7) -> (24.5, 81.4701)
  line L10 (24.5, 42.7) -> (27.5, 42.7)
  line L11 (27.5, 42.7) -> (27.5, 36.7)
  line L12 (27.5, 36.7) -> (24.5, 36.7)
  line L13 (24.5, 36.7) -> (24.5, 42.7)
  point P0 (54.1562, 233.7171)
  point P1 (27.5, 42.7)
  point P2 (24.5, 42.7)
  dimension "d48" = 6
  constraints: 16 end point, 4 parallel, 2 perpendicular, 1 collinear, 1 horizontal
  measures "d48" distance of L7.end L11.end
extrude "돌출16" cut sketch "스케치16" against normal through all contours L3 L11 L12 L13
sketch "스케치17" plane through (22.1952, -197.0171, 26.6562) normal (0, 0, 1) x (1, 0, 0)
  circle A0 centre (-19.8, 11.3) radius 5 projected
  line L0 (-13.5254, 9.7593) -> (-4.9287, 44.7701) projected
  line L1 (-34.6713, 44.7701) -> (-26.0746, 9.7593) projected
  line L2 (-13.5254, 9.7593) -> (-4.9287, 44.7701)
  line L3 (-34.6713, 44.7701) -> (-26.0746, 9.7593)
  line L4 (-53.2701, -3.5713) -> (-18.2593, 5.0254)
  line L5 (-18.2593, 17.5746) -> (-53.2701, 26.1713)
  line L6 (-4.9287, -22.1701) -> (-13.5254, 12.8407)
  line L7 (-26.0746, 12.8407) -> (-34.6713, -22.1701)
  line L8 (13.6701, 26.1713) -> (-21.3407, 17.5746)
  line L9 (-21.3407, 5.0254) -> (13.6701, -3.5713)
  line L10 (-21.5792, 4.0542) -> (13.4317, -4.5425)
  circle A1 centre (-2.5, 3.3) radius 1 projected
  line L11 (-5, -31.4) -> (-5, 6) projected
  line L12 (-5, 6) -> (0, 6) projected
  line L13 (0, 6) -> (0, -31.4) projected
  line L14 (0, -31.4) -> (-5, -31.4) projected
  circle A2 centre (-2.5, -18.7) radius 1 projected
  line L15 (-5, 6) -> (0, 6)
  line L16 (0, 6) -> (0, -1.5)
  line L17 (0, -1.5) -> (-5, -1.5)
  line L18 (-5, -1.5) -> (-5, 6)
  point P0 (-22.1952, 197.0171)
  point P1 (-18.2593, 17.5746)
  point P2 (-53.2701, 26.1713)
  point P3 (-53.2701, -3.5713)
  point P4 (-18.2593, 5.0254)
  point P5 (-26.0746, 12.8407)
  point P6 (-34.6713, -22.1701)
  point P7 (-4.9287, -22.1701)
  point P8 (-13.5254, 12.8407)
  point P9 (-21.3407, 5.0254)
  point P10 (13.6701, -3.5713)
  point P11 (13.6701, 26.1713)
  point P12 (-21.3407, 17.5746)
  dimension "d53" = 360
  dimension "d55" = 1
  dimension "d56" = 7.5
  constraints: 26 end point, 4 equal length, 2 coincident, 1 perpendicular, 43 other
  measures "d55" distance between parallel lines of L9 L10
  measures "d56" distance of L12.end L16.end
extrude "돌출17" cut sketch "스케치17" along normal up to surface (3 mm away) contours L11 L12 L13 L9 | L9 L13 L10 L11 | L10 L13 L17 L11
sketch "스케치18" plane through (22.1952, -233.7171, 54.1562) normal (1, 0, 0) x (0, 0, -1)
  circle A0 centre (17.3, 8) radius 1.35 projected
  circle A1 centre (17.3, 30) radius 1.35 projected
  line L0 (27.5, 42.7) -> (27.5, 35.2) projected
  line L1 (27.5, 35.2) -> (24.5, 35.2) projected
  line L2 (24.5, 35.2) -> (24.5, 42.7) projected
  line L3 (24.5, 42.7) -> (17.1, 42.7) projected
  arc A2 (17.1, 42.7) -> (14.6, 40.2) centre (17.1, 40.2) ccw projected
  line L4 (14.6, 40.2) -> (14.6, 8) projected
  arc A3 (14.6, 8) -> (17.3, 5.3) centre (17.3, 8) ccw projected
  line L5 (17.3, 5.3) -> (40.5, 5.3) projected
  line L6 (40.5, 42.7) -> (40.5, 5.3) projected
  line L7 (40.5, 42.7) -> (27.5, 42.7) projected
  line L8 (28, 34.7) -> (28, 42.2)
  line L9 (28, 42.2) -> (40, 42.2)
  line L10 (40, 42.2) -> (40, 5.8)
  line L11 (40, 5.8) -> (17.3, 5.8)
  arc A4 (15.1, 8) -> (17.3, 5.8) centre (17.3, 8) ccw
  line L12 (15.1, 8) -> (15.1, 40.2)
  arc A5 (17.1, 42.2) -> (15.1, 40.2) centre (17.1, 40.2) ccw
  line L13 (17.1, 42.2) -> (24, 42.2)
  line L14 (24, 42.2) -> (24, 34.7)
  line L15 (24, 34.7) -> (28, 34.7)
  line L16 (24, 42.2) -> (28, 42.2)
  line L17 (28, 42.2) -> (28, 42.7)
  line L18 (28, 42.7) -> (24, 42.7)
  line L19 (24, 42.7) -> (24, 42.2)
  point P0 (54.1562, 233.7171)
  point P1 (27.5, 42.7)
  point P2 (24, 42.7)
  point P3 (28, 42.7)
  point P4 (27.5, 42.2)
  point P5 (24.5, 42.2)
  dimension "d59" = 0.5
  constraints: 24 end point, 4 point on circle, 2 centre point, 2 parallel, 2 perpendicular, 9 other
  measures "d59" distance between parallel lines of L0 L8
extrude "돌출18" cut sketch "스케치18" against normal through all contours L7 L17 L16 L0 | L0 L16 L2 L18 | L16 L8 L15 L14 L2 L1 L0 | L2 L16 L19 L3
fillet "모깎기4" radius 1 4 edges at (19.6952, -191.0171, 26.1562) (19.6952, -191.0171, 30.1562) (19.6952, -199.0171, 30.1562) (19.6952, -199.0171, 26.1562)
sketch "스케치19" plane through (22.1952, -233.7171, 54.1562) normal (1, 0, 0) x (0, 0, -1)
  arc A0 (24, 41.7) -> (23, 42.7) centre (23, 41.7) ccw projected
  line L0 (23, 42.7) -> (17.1, 42.7) projected
  arc A1 (17.1, 42.7) -> (14.6, 40.2) centre (17.1, 40.2) ccw projected
  line L1 (14.6, 40.2) -> (14.6, 8) projected
  arc A2 (14.6, 8) -> (17.3, 5.3) centre (17.3, 8) ccw projected
  line L2 (17.3, 5.3) -> (40.5, 5.3) projected
  line L3 (40.5, 42.7) -> (40.5, 5.3) projected
  line L4 (40.5, 42.7) -> (29, 42.7) projected
  arc A3 (29, 42.7) -> (28, 41.7) centre (29, 41.7) ccw projected
  line L5 (28, 41.7) -> (28, 35.7) projected
  arc A4 (27, 34.7) -> (28, 35.7) centre (27, 35.7) ccw projected
  line L6 (27, 34.7) -> (25, 34.7) projected
  arc A5 (24, 35.7) -> (25, 34.7) centre (25, 35.7) ccw projected
  line L7 (24, 35.7) -> (24, 41.7) projected
  circle A6 centre (17.3, 30) radius 1.35 projected
  circle A7 centre (17.3, 8) radius 1.35 projected
  line L8 (40.5, 38.65) -> (40.5, 41.35) projected
  line L9 (40.5, 16.65) -> (40.5, 19.35) projected
  line L10 (40.5, 19) -> (40.5, 17) projected
  line L11 (40.5, 18) -> (40.5, 15.3)
  line L12 (40.5, 18) -> (43.2, 18) construction
  line L13 (40.5, 15.3) -> (21.1, 5.3)
  line L14 (17.3, 5.3) -> (40.5, 5.3) projected
  arc A8 (17.1, 42.7) -> (14.6, 40.2) centre (17.1, 40.2) ccw projected
  line L15 (17.1, 42.7) -> (21.1, 42.7) projected
  line L16 (21.1, 42.7) -> (21.1, 5.3) projected
  line L17 (21.1, 5.3) -> (17.3, 5.3) projected
  arc A9 (14.6, 8) -> (17.3, 5.3) centre (17.3, 8) ccw projected
  line L18 (14.6, 8) -> (14.6, 40.2) projected
  circle A10 centre (17.3, 30) radius 1.35 projected
  circle A11 centre (17.3, 8) radius 1.35 projected
  line L19 (40.5, 15.3) -> (37.5, 15.3)
  line L20 (37.5, 15.3) -> (21.1, 5.3)
  line L21 (21.1, 5.3) -> (24.1, 5.3)
  line L22 (24.1, 5.3) -> (37.5, 15.3)
  point P0 (54.1562, 233.7171)
  point P1 (40.5, 15.3)
  dimension "d63" = 2.7
  dimension "d64" = 90
  dimension "d65" = 3
  dimension "d66" = 3
  constraints: 14 end point, 2 perpendicular, 2 point on line, 1 collinear, 1 horizontal, 1 midpoint
  measures "d63" distance of L11.start L11.end
  measures "d64" angle of L11 L12
  measures "d65" distance of L11.end L19.end
  measures "d66" distance of L13.end L21.end
extrude "돌출19" cut sketch "스케치19" against normal through all contours L22 L13 L3 L2 | L22 L19 L13
sketch "스케치20" plane through (22.1952, -233.7171, 54.1562) normal (1, 0, 0) x (0, 0, -1)
  line L0 (40.5, 41) -> (40.5, 39) projected
  line L1 (40.5, 16.65) -> (40.5, 19.35) projected
  line L2 (40.5, 40) -> (40.5, 18)
  line L3 (40.5, 18) -> (35.5, 18)
  line L4 (35.5, 18) -> (35.5, 40)
  line L5 (35.5, 40) -> (40.5, 40)
  line L6 (29, 42.7) -> (40.5, 42.7) projected
  line L7 (34.5, 37.3) -> (36.5, 37.3)
  line L8 (36.5, 37.3) -> (36.5, 42.7)
  line L9 (36.5, 42.7) -> (34.5, 42.7)
  line L10 (34.5, 42.7) -> (34.5, 37.3)
  line L11 (34.5, 37.3) -> (36.5, 42.7) construction
  line L12 (36.5, 37.3) -> (34.5, 42.7) construction
  line L13 (36.5, 20.7) -> (34.5, 20.7)
  line L14 (34.5, 20.7) -> (34.5, 15.3)
  line L15 (34.5, 15.3) -> (36.5, 15.3)
  line L16 (36.5, 15.3) -> (36.5, 20.7)
  line L17 (36.5, 20.7) -> (34.5, 15.3) construction
  line L18 (34.5, 20.7) -> (36.5, 15.3) construction
  circle A0 centre (17.3, 8) radius 1.35 projected
  circle A1 centre (17.3, 30) radius 1.35 projected
  line L19 (24.1, 5.3) -> (37.5, 15.3) projected
  line L20 (37.5, 15.3) -> (40.5, 15.3) projected
  line L21 (40.5, 42.7) -> (40.5, 15.3) projected
  line L22 (40.5, 42.7) -> (29, 42.7) projected
  arc A2 (29, 42.7) -> (28, 41.7) centre (29, 41.7) ccw projected
  line L23 (28, 41.7) -> (28, 35.7) projected
  arc A3 (27, 34.7) -> (28, 35.7) centre (27, 35.7) ccw projected
  line L24 (27, 34.7) -> (25, 34.7) projected
  arc A4 (24, 35.7) -> (25, 34.7) centre (25, 35.7) ccw projected
  line L25 (24, 35.7) -> (24, 41.7) projected
  arc A5 (24, 41.7) -> (23, 42.7) centre (23, 41.7) ccw projected
  line L26 (23, 42.7) -> (17.1, 42.7) projected
  arc A6 (17.1, 42.7) -> (14.6, 40.2) centre (17.1, 40.2) ccw projected
  line L27 (14.6, 40.2) -> (14.6, 8) projected
  arc A7 (14.6, 8) -> (17.3, 5.3) centre (17.3, 8) ccw projected
  line L28 (17.3, 5.3) -> (24.1, 5.3) projected
  line L29 (34.5, 20.7) -> (36.5, 20.7)
  line L30 (36.5, 20.7) -> (36.5, 15.3)
  line L31 (36.5, 15.3) -> (34.5, 15.3)
  line L32 (34.5, 15.3) -> (34.5, 20.7)
  line L33 (36.5, 37.3) -> (34.5, 37.3)
  line L34 (34.5, 37.3) -> (34.5, 42.7)
  line L35 (34.5, 42.7) -> (36.5, 42.7)
  line L36 (36.5, 42.7) -> (36.5, 37.3)
  point P0 (54.1562, 233.7171)
  dimension "d69" = 5
  dimension "d70" = 2
  dimension "d71" = 2
  dimension "d72" = 5.4
  constraints: 48 end point, 10 parallel, 6 midpoint, 5 perpendicular, 4 horizontal, 1 point on line
  measures "d69" distance of L2.end L3.end
  measures "d70" distance of L9.end L8.end
  measures "d71" distance of L15.end L14.end
  measures "d72" distance of L14.end L13.end
extrude "돌출20" cut sketch "스케치20" against normal through all contours L8 L7 L4 L5 | L5 L4 L7 L10 L6 L8 | L16 L15 L14 L13 L4 L3 | L3 L4 L13 L16
sketch "스케치21" plane through (22.1952, -233.7171, 54.1562) normal (1, 0, 0) x (0, 0, -1)
  line L0 (34.5, 37.3) -> (34.5, 42.7) projected
  line L1 (34.5, 42.7) -> (29, 42.7) projected
  arc A0 (29, 42.7) -> (28, 41.7) centre (29, 41.7) ccw projected
  line L2 (28, 41.7) -> (28, 35.7) projected
  arc A1 (27, 34.7) -> (28, 35.7) centre (27, 35.7) ccw projected
  line L3 (27, 34.7) -> (25, 34.7) projected
  arc A2 (24, 35.7) -> (25, 34.7) centre (25, 35.7) ccw projected
  line L4 (24, 35.7) -> (24, 41.7) projected
  arc A3 (24, 41.7) -> (23, 42.7) centre (23, 41.7) ccw projected
  line L5 (23, 42.7) -> (17.1, 42.7) projected
  arc A4 (17.1, 42.7) -> (14.6, 40.2) centre (17.1, 40.2) ccw projected
  line L6 (14.6, 40.2) -> (14.6, 8) projected
  arc A5 (14.6, 8) -> (17.3, 5.3) centre (17.3, 8) ccw projected
  line L7 (17.3, 5.3) -> (24.1, 5.3) projected
  line L8 (24.1, 5.3) -> (37.5, 15.3) projected
  line L9 (37.5, 15.3) -> (40.5, 15.3) projected
  line L10 (40.5, 42.7) -> (40.5, 15.3) projected
  line L11 (40.5, 42.7) -> (36.5, 42.7) projected
  line L12 (36.5, 42.7) -> (36.5, 37.3) projected
  line L13 (36.5, 37.3) -> (34.5, 37.3) projected
  line L14 (34.5, 15.3) -> (34.5, 20.7) projected
  line L15 (34.5, 20.7) -> (36.5, 20.7) projected
  line L16 (36.5, 20.7) -> (36.5, 15.3) projected
  line L17 (36.5, 15.3) -> (34.5, 15.3) projected
  circle A6 centre (17.3, 8) radius 1.35 projected
  circle A7 centre (17.3, 30) radius 1.35 projected
  line L18 (40.5, 15.3) -> (34.5, 15.3)
  line L19 (24.1, 5.3) -> (34.5, 15.3)
  point P0 (54.1562, 233.7171)
  constraints: 4 end point, 1 perpendicular
extrude "돌출21" cut sketch "스케치21" against normal through all contours L8 L19 L17 L18
fillet "모깎기5" radius 1 4 edges at (19.6952, -218.4171, 19.6562) (19.6952, -218.4171, 17.6562) (19.6952, -191.0171, 19.6562) (19.6952, -191.0171, 17.6562)
equation "\"TransitionRadius\" = BendRadius"
equation "\"BendRadius\" = 0.5"
